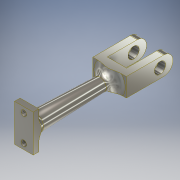
# Autodesk Inventor part: reverse gear crank rod 1
Saved by Autodesk Inventor 2017 (Build 210142000, 142)
## iProperties
Created: 2018-11-07
Part Number: reverse gear crank rod 1
Material: Generic
Document SubType Name: Modeling
Designer: User
Density: 1 g/cm^3
Appearance: Default
Author: User
Autodesk Inventor part; units mm, degrees
ref_plane "XY Plane" through (0, 0, 0) normal (0, 0, 1) x (1, 0, 0)
sketch "Sketch1" plane through (0, 0, 0) normal (0, 1, 0) x (-1, 0, 0)
  circle A0 centre (0, 0) radius 4.75
  dimension "d0" = 9.5
  dimension "d31" = 0
  constraints: 1 centre point, 1 coincident
  measures "d0" diameter of A0
  measures "d31" distance of point (0, 0) A0.centre
ref_plane "Work Plane1" through (0, 43, 0) normal (0, 1, 0) x (-1, 0, 0)
sketch "Sketch2" plane through (0, 43, 0) normal (0, 1, 0) x (-1, 0, 0)
  circle A0 centre (0, 0) radius 3.25
  dimension "d2" = 6.5
  dimension "d32" = 0
  constraints: 1 centre point, 1 coincident
  measures "d2" diameter of A0
  measures "d32" distance of point (0, 0) A0.centre
loft "Loft1" add profiles "Sketch1", "Sketch2"
sketch "Sketch3" plane through (0, 0, 0) normal (0, -1, 0) x (1, 0, 0)
  circle A0 centre (0, 0) radius 4.75
  line L0 (0, 0) -> (5, 0)
  line L1 (5, 0) -> (5, -10)
  line L2 (5, -10) -> (-5, -10)
  line L3 (-5, -10) -> (-5, 10)
  line L4 (-5, 10) -> (5, 10)
  line L5 (5, 10) -> (5, 0)
  dimension "d7" = 5
  dimension "d8" = 10
  dimension "d9" = 10
  dimension "d10" = 20
  dimension "d11" = 10
  dimension "d33" = 9.5
  dimension "d34" = 5
  dimension "d35" = 0
  dimension "d36" = 5
  dimension "d37" = 0
  constraints: 12 end point, 3 perpendicular, 1 centre point, 1 horizontal, 1 point on line
  measures "d7" distance of L0.start L0.end
  measures "d8" distance of L0.end L1.end
  measures "d9" distance of L1.end L2.end
  measures "d10" distance of L2.end L3.end
  measures "d11" distance of L3.end L4.end
  measures "d33" diameter of A0
  measures "d34" distance from line of point (0, 0) L1
  measures "d35" distance from line of point (0, 0) L0
  measures "d36" distance from line of point (0, 0) L1
  measures "d37" distance from line of point (0, 0) L0
extrude "Extrusion1" add sketch "Sketch3" along normal blind 3
sketch "Sketch4" plane through (0, 0, 0) normal (0, -1, 0) x (1, 0, 0)
  circle A0 centre (0, 0) radius 5
  dimension "d14" = 10
  dimension "d38" = 0
  constraints: 1 centre point, 1 coincident
  measures "d14" diameter of A0
  measures "d38" distance of point (0, 0) A0.centre
extrude "Extrusion2" add sketch "Sketch4" along normal blind 3
sketch "Sketch5" plane through (0, 0, 0) normal (0, 1, 0) x (1, 0, 0)
  line L0 (-5, -10) -> (5, -10)
  line L1 (0, -10) -> (0, -7)
  line L2 (0, -7) -> (0, 7)
  circle A0 centre (0, -7) radius 1.5
  circle A1 centre (0, 7) radius 1.5
  point P0 (0, 0)
  point P1 (0, 0)
  dimension "d17" = 3
  dimension "d18" = 14
  dimension "d19" = 3
  dimension "d20" = 3
  dimension "d39" = 0
  dimension "d40" = 10
  dimension "d41" = 5
  dimension "d42" = 0
  dimension "d43" = 10
  constraints: 6 end point, 2 centre point, 2 coincident, 1 horizontal, 1 midpoint, 1 point on line, 1 vertical
  measures "d17" distance of L1.start L1.end
  measures "d18" distance of L1.end L2.end
  measures "d19" diameter of A0
  measures "d20" diameter of A1
  measures "d39" distance from line of point (0, 0) L1
  measures "d40" distance from line of point (0, 0) L0
  measures "d41" distance from line of L0.end L1
  measures "d42" distance from line of point (0, 0) L1
  measures "d43" distance from line of point (0, 0) L0
extrude "Extrusion3" cut sketch "Sketch5" against normal through all
fillet "Fillet1" radius 3 1 edges at (4.75, 0, 0)
sketch "Sketch7" plane through (0, 43, 0) normal (0, 1, 0) x (1, 0, 0)
  line L0 (0, 0) -> (5, 0) construction
  line L1 (5, 0) -> (-5, 0) construction
  line L2 (-5, 0) -> (-5, -9) construction
  line L3 (9, 4.5) -> (-9, 4.5)
  line L4 (-9, 4.5) -> (-9, -5.5)
  line L5 (9, 4.5) -> (9, -5.5)
  line L6 (9, -5.5) -> (-9, -5.5)
  point P0 (-5, 9)
  dimension "d79" = 10
  dimension "d80" = 4.5
  dimension "d81" = 10
  dimension "d82" = 14
  dimension "d83" = 18
  dimension "d84" = 9
  dimension "d85" = 4
  dimension "d86" = 9
  dimension "d87" = 9
  constraints: 14 end point, 2 horizontal, 2 perpendicular, 2 point on line, 1 vertical
  measures "d79" distance of L3.end L4.end
  measures "d80" distance between parallel lines of L1 L3
  measures "d81" distance of L3.start L5.end
  measures "d82" distance between parallel lines of L2 L5
  measures "d83" distance between parallel lines of L5 L4
  measures "d84" distance from line of L0.start L5
  measures "d85" distance from line of L0.end L5
  measures "d86" distance from line of point (-5, 9) L0
  measures "d87" distance from line of L2.end L0
extrude "Extrusion5" add sketch "Sketch7" along normal blind 4
fillet "Fillet4" radius 5 1 edges at (3.25, 43, 0)
sketch "Sketch10" plane through (0, 47, 0) normal (0, 1, 0) x (1, 0, 0)
  line L0 (-9, -5.5) -> (9, -5.5) projected
  line L1 (5.1815, -5.5) -> (5.1564, 4.5)
  line L2 (9, 4.5) -> (-9, 4.5) projected
  line L3 (9, 4.5) -> (5.1564, 4.5)
  line L4 (9, -5.5) -> (9, 4.5)
  line L5 (9, -5.5) -> (5.1815, -5.5)
  point P0 (0, 0)
  constraints: 8 end point, 2 perpendicular, 2 point on line, 1 collinear
extrude "Extrusion8" add sketch "Sketch10" along normal blind 21
fillet "Fillet5" radius 5 2 edges at (7.0782, 68, -4.5) (7.0907, 68, 5.5)
sketch "Sketch11" plane through (5.1564, 47, -4.5) normal (-0.9999968, 0, 0.002511) x (0.002511, 0, 0.9999968)
  circle A0 centre (5, 14.0634) radius 3
  line L0 (10, 0) -> (10, 16) projected
  line L1 (0, 0) -> (0, 16) projected
  point P0 (4.487, -47)
  dimension "d92" = 6
  dimension "d93" = 5
  dimension "d94" = 5.3619
  constraints: 1 centre point
  measures "d92" diameter of A0
  measures "d93" distance from line of L0 A0.centre
  measures "d94" distance of L0.end A0.centre
extrude "Extrusion9" cut sketch "Sketch11" against normal blind 21
ref_plane "Work Plane2" through (0, 0, 0) normal (1, 0, 0) x (0, 1, 0)
mirror "Mirror1" about plane through (0, 0, 0) normal (1, 0, 0)
body "Solid1"
